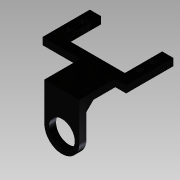
# Autodesk Inventor part: Dudukan Proximity Servo
Saved by Autodesk Inventor 2015 SP1 (Build 190203100, 203)
## iProperties
Created: 2015-02-11
Part Number: Dudukan Proximity Servo
Material: Generic
Document SubType Name: Modeling
Designer: Rafi Kurnia Putra
Density: 1 g/cm^3
Appearance: Smooth - Purple
Author: Rafi Kurnia Putra
Autodesk Inventor part; units mm, degrees
ref_plane "XZ Plane" through (0, 0, 0) normal (0, 1, 0) x (-1, 0, 0)
sketch "Sketch1" plane through (0, 0, 0) normal (0, 1, 0) x (-1, 0, 0)
  circle A0 centre (24.5999, -4.9022) radius 2.2225
  line L0 (26.4238, -3.6322) -> (26.6065, -3.6322)
  circle A1 centre (24.5999, 4.9022) radius 2.2225
  line L1 (26.6196, 9.4615) -> (23.1196, 9.4615)
  line L2 (26.6065, -9.4615) -> (20.6065, -9.4615)
  line L3 (26.4238, -6.1722) -> (26.6065, -6.1722)
  line L4 (23.1196, 9.4615) -> (23.1196, 14.4615)
  line L5 (-26.4238, -3.6322) -> (-26.6065, -3.6322)
  line L6 (-26.4238, -6.1722) -> (-26.6065, -6.1722)
  line L7 (-26.6065, -9.4615) -> (-20.6065, -9.4615)
  circle A2 centre (-24.5999, -4.9022) radius 2.2225
  circle A3 centre (-24.5999, 4.9022) radius 2.2225
  line L8 (-26.6196, 9.4615) -> (-23.1196, 9.4615)
  line L9 (-23.1196, 9.4615) -> (-23.1196, 14.4615)
  line L10 (20.6065, 10.9615) -> (-20.6065, 10.9615)
  line L11 (23.1196, 14.4615) -> (21.9202, 14.4615)
  line L12 (-12.375, 14.4615) -> (-23.1196, 14.4615)
  line L13 (21.9202, 14.4593) -> (21.9202, 39.4593)
  line L14 (21.9202, 14.4593) -> (46.9202, 14.4593) construction
  line L15 (21.9202, 39.4593) -> (-2.8298, 39.4615)
  line L16 (-2.8298, 39.4615) -> (-2.832, 14.4615)
  line L17 (-2.832, 14.4615) -> (-12.375, 14.4615)
  line L18 (-26.6196, 9.4615) -> (-29.5802, 9.4615)
  line L19 (-29.5802, 9.4615) -> (-29.5802, -9.4615)
  line L20 (-29.5802, -9.4615) -> (-26.6065, -9.4615)
  line L21 (26.6196, 9.4615) -> (29.5802, 9.4615)
  line L22 (29.5802, 9.4615) -> (29.5802, -9.4615)
  line L23 (29.5802, -9.4615) -> (26.6065, -9.4615)
  line L24 (-20.6065, -9.4615) -> (-20.6065, 10.9615)
  line L25 (20.6065, -9.4615) -> (20.6065, 10.9615)
  point P0 (-26.4238, 3.6322)
  point P1 (0, 0)
  point P2 (9.5452, 14.4593)
  dimension "d38" = 90
  dimension "d39" = 24.75
  dimension "d41" = 90
  dimension "d43" = 4.9803
  dimension "d45" = 4.9803
  constraints: 52 end point, 6 horizontal, 4 perpendicular, 4 point on circle, 3 centre point, 3 vertical, 1 collinear, 1 parallel, 1 point on line, 4 other
  measures "d38" angle of L14 L13
  measures "d39" distance of L13.end L15.end
  measures "d41" angle of L16 L15
  measures "d43" horizontal distance of L18.end point (-24.6, 4.902)
  measures "d45" horizontal distance of L21.end A1.centre
extrude "Extrusion1" add sketch "Sketch1" along normal blind 3 contours A0 | A1 | L21 L22 L23 L2 L25 L10 L24 L7 L20 L19 L18 L8 L9 L12 L17 L16 L15 L13 L11 L4 L1 | A2 | A3
ref_plane "Work Plane1" through (0, 0, 39.4615) normal (0, 0, 1) x (1, 0, 0)
sketch "Sketch2" plane through (0, 0, 39.4615) normal (0, 0, 1) x (1, 0, 0)
  circle A0 centre (-9.5452, 25) radius 9.125
  line L0 (-21.9202, 0) -> (2.8298, 0)
  arc A1 (2.8298, 25) -> (-21.9202, 25) centre (-9.5452, 25) ccw
  line L1 (2.8298, 0) -> (2.8298, 25)
  line L2 (-21.9202, 0) -> (-21.9202, 25)
  point P0 (0, 0)
  point P1 (-9.5452, 0)
  dimension "d23" = 18.25
  dimension "d24" = 24.75
  dimension "d25" = 24.75
  dimension "d26" = 25
  dimension "d27" = 25
  constraints: 6 end point, 2 centre point, 2 coincident, 2 horizontal, 2 point on circle, 2 tangent, 1 midpoint
  measures "d23" diameter of A0
  measures "d24" diameter of A1
  measures "d25" distance of L0.start L0.end
  measures "d26" distance of L0.start L2.end
  measures "d27" distance of L0.end L1.end
extrude "Extrusion2" add sketch "Sketch2" along normal blind 3
extrude "Extrusion3" cut sketch "Sketch1" along normal up to next contours A0 | A1 | A2 | A3
sketch "Sketch3" plane through (0, 0, 0) normal (0, -1, 0) x (1, 0, 0)
  circle A0 centre (-24.5999, -4.9022) radius 2.2225 projected
  circle A1 centre (-24.5999, 4.9022) radius 2.2225 projected
  circle A2 centre (24.5999, 4.9022) radius 2.2225 projected
  circle A3 centre (24.5999, -4.9022) radius 2.2225 projected
  line L0 (-29.5802, -9.4615) -> (-20.6065, -9.4615) projected
  line L1 (-20.6065, -9.4615) -> (-20.6065, 10.9615) projected
  line L2 (-20.6065, 10.9615) -> (20.6065, 10.9615) projected
  line L3 (20.6065, 10.9615) -> (20.6065, -9.4615) projected
  line L4 (20.6065, -9.4615) -> (29.5802, -9.4615) projected
  line L5 (29.5802, -9.4615) -> (29.5802, 9.4615) projected
  line L6 (29.5802, 9.4615) -> (23.1196, 9.4615) projected
  line L7 (23.1196, 9.4615) -> (23.1196, 14.4615) projected
  line L8 (23.1196, 14.4615) -> (2.832, 14.4615) projected
  line L9 (2.832, 14.4615) -> (2.8298, 39.4615) projected
  line L10 (2.8298, 39.4615) -> (-21.9202, 39.4593) projected
  line L11 (-21.9202, 39.4593) -> (-21.9202, 14.4615) projected
  line L12 (-21.9202, 14.4615) -> (-23.1196, 14.4615) projected
  line L13 (-23.1196, 14.4615) -> (-23.1196, 9.4615) projected
  line L14 (-23.1196, 9.4615) -> (-29.5802, 9.4615) projected
  line L15 (-29.5802, 9.4615) -> (-29.5802, -9.4615) projected
  line L16 (-21.9202, 39.4615) -> (2.8298, 39.4615) projected
  line L17 (2.8298, 39.4615) -> (2.8298, 42.4615) projected
  line L18 (-21.9202, 42.4615) -> (2.8298, 42.4615) projected
  line L19 (-21.9202, 39.4615) -> (-21.9202, 42.4615) projected
  point P0 (0, 0)
extrude "Extrusion4" add sketch "Sketch3" along normal blind 2
sketch "Sketch4" plane through (0, -2, 0) normal (0, -1, 0) x (1, 0, 0)
  circle A0 centre (24.5999, -4.9022) radius 2.2225 projected
  circle A1 centre (24.5999, 4.9022) radius 2.2225 projected
  circle A2 centre (-24.5999, 4.9022) radius 2.2225 projected
  circle A3 centre (-24.5999, -4.9022) radius 2.2225 projected
  line L0 (-29.5802, -9.4615) -> (-20.6065, -9.4615) projected
  line L1 (-20.6065, -9.4615) -> (-20.6065, 10.9615) projected
  line L2 (-20.6065, 10.9615) -> (20.6065, 10.9615) projected
  line L3 (20.6065, 10.9615) -> (20.6065, -9.4615) projected
  line L4 (20.6065, -9.4615) -> (29.5802, -9.4615) projected
  line L5 (29.5802, -9.4615) -> (29.5802, 9.4615) projected
  line L6 (29.5802, 9.4615) -> (23.1196, 9.4615) projected
  line L7 (23.1196, 9.4615) -> (23.1196, 14.4615) projected
  line L8 (23.1196, 14.4615) -> (2.832, 14.4615) projected
  line L9 (2.832, 14.4615) -> (2.8298, 39.4615) projected
  line L10 (2.8298, 39.4615) -> (-21.9202, 39.4593) projected
  line L11 (-21.9202, 39.4593) -> (-21.9202, 14.4615) projected
  line L12 (-21.9202, 14.4615) -> (-23.1196, 14.4615) projected
  line L13 (-23.1196, 14.4615) -> (-23.1196, 9.4615) projected
  line L14 (-23.1196, 9.4615) -> (-29.5802, 9.4615) projected
  line L15 (-29.5802, 9.4615) -> (-29.5802, -9.4615) projected
  line L16 (2.832, 14.4615) -> (23.1196, 14.4615)
  line L17 (23.1196, 14.4615) -> (23.1196, 16.4615)
  line L18 (23.1196, 16.4615) -> (2.832, 16.4615)
  line L19 (2.832, 16.4615) -> (2.832, 14.4615)
  line L20 (-21.9202, 14.4615) -> (-23.1196, 14.4615)
  line L21 (-23.1196, 14.4615) -> (-23.1196, 16.4615)
  line L22 (-23.1196, 16.4615) -> (-21.9202, 16.4615)
  line L23 (-21.9202, 16.4615) -> (-21.9202, 14.4615)
  point P0 (0, 0)
  dimension "d52" = 2
  dimension "d53" = 2
  constraints: 16 end point, 4 parallel, 2 horizontal, 2 perpendicular
  measures "d52" distance of L17.end L16.end
  measures "d53" distance of L20.end L21.end
extrude "Extrusion5" add sketch "Sketch4" against normal blind 5 contours L21 L22 L11 L12 | L8 L9 L18 L17
sketch "Sketch5" plane through (0, -2, 0) normal (0, -1, 0) x (1, 0, 0)
  line L0 (20.6065, 10.9615) -> (-20.6065, 10.9615)
  line L1 (-20.6065, 10.9615) -> (-20.6065, 11.9615)
  line L2 (-20.6065, 11.9615) -> (20.6065, 11.9615)
  line L3 (20.6065, 11.9615) -> (20.6065, 10.9615)
  point P0 (0, 0)
  dimension "d56" = 1
  constraints: 8 end point, 2 parallel, 1 horizontal, 1 perpendicular
  measures "d56" distance of L0.end L1.end
extrude "Extrusion6" cut sketch "Sketch5" against normal up to next
sketch "Sketch6" plane through (0, -2, 0) normal (0, -1, 0) x (1, 0, 0)
  line L0 (21.6065, 11.9615) -> (-21.6065, 11.9615)
  line L1 (-21.6065, 11.9615) -> (-21.6065, -9.4615)
  line L2 (-21.6065, -9.4615) -> (21.6065, -9.4615)
  line L3 (21.6065, -9.4615) -> (21.6065, 11.9615)
  line L4 (20.6065, 11.9615) -> (20.6065, -9.4615) projected
  line L5 (-20.6065, -9.4615) -> (-20.6065, 11.9615) projected
  line L6 (-20.6065, 11.9615) -> (20.6065, 11.9615) projected
  point P0 (0, 0)
  dimension "d59" = 1
  dimension "d60" = 1
  dimension "d61" = 0
  constraints: 8 end point, 2 parallel, 1 horizontal, 1 perpendicular
  measures "d59" distance between parallel lines of L3 L4
  measures "d60" distance between parallel lines of L1 L5
  measures "d61" distance between parallel lines of L0 L6
extrude "Extrusion7" cut sketch "Sketch6" against normal up to next
sketch "Sketch7" plane through (0, -2, 0) normal (0, -1, 0) x (1, 0, 0)
  line L0 (-23.1196, 9.4615) -> (-29.5802, 9.4615)
  line L1 (-29.5802, 9.4615) -> (-29.5802, 16.4615)
  line L2 (-29.5802, 16.4615) -> (-23.1196, 16.4615)
  line L3 (-23.1196, 16.4615) -> (-23.1196, 9.4615)
  line L4 (23.1196, 9.4615) -> (29.5802, 9.4615)
  line L5 (29.5802, 9.4615) -> (29.5802, 16.4615)
  line L6 (29.5802, 16.4615) -> (23.1196, 16.4615)
  line L7 (23.1196, 16.4615) -> (23.1196, 9.4615)
  point P0 (0, 0)
  dimension "d64" = 7
  dimension "d65" = 6.4606
  constraints: 16 end point, 4 parallel, 2 horizontal, 2 perpendicular
  measures "d64" distance of L0.end L1.end
  measures "d65" distance of L1.end L2.end
extrude "Extrusion8" add sketch "Sketch7" against normal blind 5
sketch "Sketch8" plane through (0, -2, 0) normal (0, -1, 0) x (1, 0, 0)
  line L0 (-29.5802, -9.4615) -> (-21.6062, -9.4615)
  line L1 (-21.6062, -9.4615) -> (-21.6062, -14.4615)
  line L2 (-21.6062, -14.4615) -> (-29.5802, -14.4615)
  line L3 (-29.5802, -14.4615) -> (-29.5802, -9.4615)
  point P0 (0, 0)
  dimension "d68" = 7.974
  dimension "d69" = 5
  constraints: 8 end point, 2 parallel, 1 horizontal, 1 perpendicular
  measures "d68" distance of L1.end L2.end
  measures "d69" distance of L0.end L1.end
extrude "Extrusion9" add sketch "Sketch8" against normal blind 5
mirror "Mirror1" about plane through (0, 0, 0) normal (1, 0, 0) of "Extrusion9"
sketch "Sketch9" plane through (0, -2, 0) normal (0, -1, 0) x (1, 0, 0)
  line L0 (-29.5802, -14.4615) -> (-29.5802, 16.4615) projected
  line L1 (-29.5802, 12) -> (29.5798, 12)
  line L2 (29.5798, 12) -> (29.5798, 19)
  line L3 (29.5798, 19) -> (-29.5802, 19)
  line L4 (-29.5802, 19) -> (-29.5802, 12)
  point P0 (0, 0)
  dimension "d72" = 59.16
  constraints: 8 end point, 2 parallel, 1 horizontal, 1 perpendicular, 1 point on line
  measures "d72" distance of L3.end L2.end
extrude "Extrusion10" add sketch "Sketch9" against normal blind 5
sketch "Sketch10" plane through (0, 0, 42.4615) normal (0, 0, 1) x (1, 0, 0)
  circle A0 centre (-9.5452, 25) radius 9.125 projected
  line L0 (2.8298, 0) -> (2.8298, 25) projected
  arc A1 (2.8298, 25) -> (-21.9202, 25) centre (-9.5452, 25) ccw projected
  line L1 (-21.9202, 25) -> (-21.9202, -2) projected
  line L2 (2.8298, -2) -> (-21.9202, -2) projected
  line L3 (2.8298, 0) -> (2.8298, -2) projected
  point P0 (0, 0)
extrude "Extrusion11" add sketch "Sketch10" along normal blind 2
ref_plane "Work Plane2" through (-9.545, 0, 0) normal (1, 0, 0) x (0, 1, 0)
sketch "Sketch12" plane through (-9.545, 0, 0) normal (1, 0, 0) x (0, 1, 0)
  line L0 (3, 39.4615) -> (8, 39.4615)
  line L1 (8, 39.4615) -> (3, 34.4615)
  line L2 (3, 34.4615) -> (3, 39.4615)
  line L3 (3, 39.4615) -> (8, 39.4615)
  line L4 (3, 39.4615) -> (25, 39.4615) projected
  point P0 (0, 0)
  dimension "d79" = 5
  dimension "d80" = 45
  dimension "d83" = 5
  constraints: 8 end point, 1 collinear, 1 horizontal, 1 vertical
  measures "d79" distance of L0.start L0.end
  measures "d80" angle of L0 L1
  measures "d83" distance of L1.end L2.end
extrude "Extrusion12" add sketch "Sketch12" along normal mid plane 24.75
equation "\"d43\" = d42"
equation "\"d45\" = d44"
equation "\"d27\" = d26"
equation "\"d44\" = 4.980307"
equation "\"d42\" = 4.980307"
body "Solid1"
